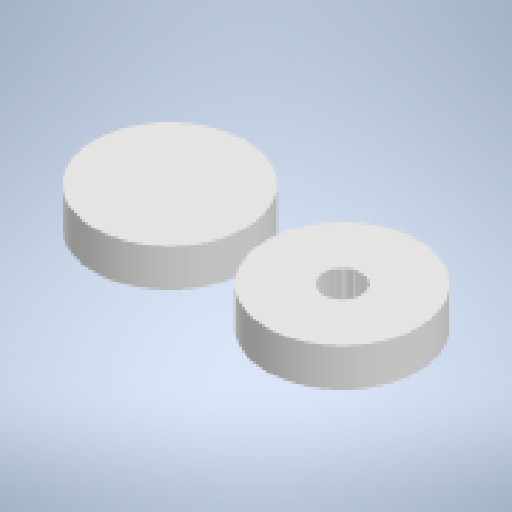
# Autodesk Inventor part: klesce2
Saved by Autodesk Inventor 2024 (Build 280153000, 153)
## iProperties
Created: 2023-09-14
Part Number: klesce2
Material: Generic
Document SubType Name: Modeling
Designer: jebes windows
Density: 1 g/cm^3
Appearance: Default
Author: jebes windows
Autodesk Inventor part; units mm, degrees
ref_plane "YZ Plane" through (0, 0, 0) normal (1, 0, 0) x (0, 1, 0)
ref_plane "XZ Plane" through (0, 0, 0) normal (0, 1, 0) x (-1, 0, 0)
ref_plane "XY Plane" through (0, 0, 0) normal (0, 0, 1) x (1, 0, 0)
sketch "Sketch1" plane through (0, 0, 0) normal (0, 0, 1) x (1, 0, 0)
  circle A0 centre (0, 0) radius 2.25 projected
  circle A1 centre (0, 0) radius 0.8 projected
  line L0 (-1.3596, 2.0381) -> (-1.3813, 1.9012) projected
  arc A2 (-1.3089, 2.071) -> (-1.3596, 2.0381) centre (0, 0) ccw projected
  line L1 (-1.175, 2.0352) -> (-1.3089, 2.071) projected
  line L2 (-1.1391, 2.1691) -> (-1.175, 2.0352) projected
  arc A3 (-1.0853, 2.1965) -> (-1.1391, 2.1691) centre (0, 0) ccw projected
  line L3 (-0.9558, 2.1468) -> (-1.0853, 2.1965) projected
  circle A4 centre (0, 0) radius 2.5 projected
  circle A5 centre (0, 0) radius 0.8 projected
  line L4 (-0.9061, 2.2763) -> (-0.9558, 2.1468) projected
  arc A6 (-0.8497, 2.2979) -> (-0.9061, 2.2763) centre (0, 0) ccw projected
  line L5 (-0.7262, 2.235) -> (-0.8497, 2.2979) projected
  line L6 (-0.6632, 2.3585) -> (-0.7262, 2.235) projected
  arc A7 (-0.6049, 2.3742) -> (-0.6632, 2.3585) centre (0, 0) ccw projected
  line L7 (-0.4886, 2.2986) -> (-0.6049, 2.3742) projected
  line L8 (-0.4131, 2.4149) -> (-0.4886, 2.2986) projected
  arc A8 (-0.3534, 2.4244) -> (-0.4131, 2.4149) centre (0, 0) ccw projected
  line L9 (-0.2456, 2.3371) -> (-0.3534, 2.4244) projected
  line L10 (-0.1584, 2.4449) -> (-0.2456, 2.3371) projected
  arc A9 (-0.098, 2.448) -> (-0.1584, 2.4449) centre (0, 0) ccw projected
  line L11 (0, 2.35) -> (-0.098, 2.448) projected
  line L12 (-1.5652, 1.8848) -> (-1.5725, 1.7464) projected
  line L13 (-1.3813, 1.9012) -> (-1.5182, 1.9229) projected
  arc A10 (-1.5182, 1.9229) -> (-1.5652, 1.8848) centre (0, 0) ccw projected
  line L14 (-1.5725, 1.7464) -> (-1.7109, 1.7536) projected
  arc A11 (-1.7109, 1.7536) -> (-1.7536, 1.7109) centre (0, 0) ccw projected
  line L15 (-1.7536, 1.7109) -> (-1.7464, 1.5725) projected
  line L16 (-1.7464, 1.5725) -> (-1.8848, 1.5652) projected
  arc A12 (-1.8848, 1.5652) -> (-1.9229, 1.5182) centre (0, 0) ccw projected
  line L17 (-1.9229, 1.5182) -> (-1.9012, 1.3813) projected
  line L18 (-1.9012, 1.3813) -> (-2.0381, 1.3596) projected
  arc A13 (-2.0381, 1.3596) -> (-2.071, 1.3089) centre (0, 0) ccw projected
  line L19 (-2.071, 1.3089) -> (-2.0352, 1.175) projected
  line L20 (-2.0352, 1.175) -> (-2.1691, 1.1391) projected
  arc A14 (-2.1691, 1.1391) -> (-2.1965, 1.0853) centre (0, 0) ccw projected
  line L21 (-2.1965, 1.0853) -> (-2.1468, 0.9558) projected
  circle A15 centre (0, 0) radius 2.5 projected
  circle A16 centre (0, 0) radius 0.8 projected
  line L22 (-2.1468, 0.9558) -> (-2.2763, 0.9061) projected
  arc A17 (-2.2763, 0.9061) -> (-2.2979, 0.8497) centre (0, 0) ccw projected
  line L23 (-2.2979, 0.8497) -> (-2.235, 0.7262) projected
  line L24 (-2.235, 0.7262) -> (-2.3585, 0.6632) projected
  arc A18 (-2.3585, 0.6632) -> (-2.3742, 0.6049) centre (0, 0) ccw projected
  line L25 (-2.3742, 0.6049) -> (-2.2986, 0.4886) projected
  line L26 (-2.2986, 0.4886) -> (-2.4149, 0.4131) projected
  arc A19 (-2.4149, 0.4131) -> (-2.4244, 0.3534) centre (0, 0) ccw projected
  circle A20 centre (0, 0) radius 2.5 projected
  circle A21 centre (0, 0) radius 0.8 projected
  line L27 (-2.4244, 0.3534) -> (-2.3371, 0.2456) projected
  circle A22 centre (0, 0) radius 2.5 projected
  circle A23 centre (0, 0) radius 0.8 projected
  line L28 (-2.3371, 0.2456) -> (-2.4449, 0.1584) projected
  arc A24 (-2.4449, 0.1584) -> (-2.448, 0.098) centre (0, 0) ccw projected
  circle A25 centre (0, 0) radius 2.5 projected
  circle A26 centre (0, 0) radius 0.8 projected
  line L29 (-2.448, 0.098) -> (-2.35, 0) projected
  line L30 (0.098, 2.448) -> (0, 2.35) projected
  arc A27 (0.1584, 2.4449) -> (0.098, 2.448) centre (0, 0) ccw projected
  line L31 (0.2456, 2.3371) -> (0.1584, 2.4449) projected
  line L32 (0.3534, 2.4244) -> (0.2456, 2.3371) projected
  arc A28 (0.4131, 2.4149) -> (0.3534, 2.4244) centre (0, 0) ccw projected
  line L33 (0.4886, 2.2986) -> (0.4131, 2.4149) projected
  line L34 (0.6049, 2.3742) -> (0.4886, 2.2986) projected
  line L35 (0.7262, 2.235) -> (0.6632, 2.3585) projected
  arc A29 (0.6632, 2.3585) -> (0.6049, 2.3742) centre (0, 0) ccw projected
  line L36 (0.8497, 2.2979) -> (0.7262, 2.235) projected
  line L37 (0.9558, 2.1468) -> (0.9061, 2.2763) projected
  arc A30 (0.9061, 2.2763) -> (0.8497, 2.2979) centre (0, 0) ccw projected
  line L38 (1.0853, 2.1965) -> (0.9558, 2.1468) projected
  line L39 (1.175, 2.0352) -> (1.1391, 2.1691) projected
  arc A31 (1.1391, 2.1691) -> (1.0853, 2.1965) centre (0, 0) ccw projected
  line L40 (1.3089, 2.071) -> (1.175, 2.0352) projected
  arc A32 (1.3596, 2.0381) -> (1.3089, 2.071) centre (0, 0) ccw projected
  line L41 (1.3813, 1.9012) -> (1.3596, 2.0381) projected
  line L42 (1.5182, 1.9229) -> (1.3813, 1.9012) projected
  arc A33 (1.5652, 1.8848) -> (1.5182, 1.9229) centre (0, 0) ccw projected
  line L43 (1.5725, 1.7464) -> (1.5652, 1.8848) projected
  line L44 (1.7109, 1.7536) -> (1.5725, 1.7464) projected
  line L45 (1.7464, 1.5725) -> (1.7536, 1.7109) projected
  arc A34 (1.7536, 1.7109) -> (1.7109, 1.7536) centre (0, 0) ccw projected
  line L46 (1.8848, 1.5652) -> (1.7464, 1.5725) projected
  arc A35 (1.9229, 1.5182) -> (1.8848, 1.5652) centre (0, 0) ccw projected
  line L47 (1.9012, 1.3813) -> (1.9229, 1.5182) projected
  line L48 (2.0381, 1.3596) -> (1.9012, 1.3813) projected
  arc A36 (2.071, 1.3089) -> (2.0381, 1.3596) centre (0, 0) ccw projected
  line L49 (2.0352, 1.175) -> (2.071, 1.3089) projected
  line L50 (2.1691, 1.1391) -> (2.0352, 1.175) projected
  arc A37 (2.1965, 1.0853) -> (2.1691, 1.1391) centre (0, 0) ccw projected
  line L51 (2.1468, 0.9558) -> (2.1965, 1.0853) projected
  line L52 (2.2763, 0.9061) -> (2.1468, 0.9558) projected
  circle A38 centre (0, 0) radius 2.5 projected
  circle A39 centre (0, 0) radius 0.8 projected
  arc A40 (2.2979, 0.8497) -> (2.2763, 0.9061) centre (0, 0) ccw projected
  line L53 (2.235, 0.7262) -> (2.2979, 0.8497) projected
  line L54 (2.3585, 0.6632) -> (2.235, 0.7262) projected
  arc A41 (2.3742, 0.6049) -> (2.3585, 0.6632) centre (0, 0) ccw projected
  line L55 (2.2986, 0.4886) -> (2.3742, 0.6049) projected
  line L56 (2.4149, 0.4131) -> (2.2986, 0.4886) projected
  circle A42 centre (0, 0) radius 2.5 projected
  circle A43 centre (0, 0) radius 0.8 projected
  arc A44 (2.4244, 0.3534) -> (2.4149, 0.4131) centre (0, 0) ccw projected
  circle A45 centre (0, 0) radius 2.5 projected
  circle A46 centre (0, 0) radius 0.8 projected
  line L57 (2.3371, 0.2456) -> (2.4244, 0.3534) projected
  line L58 (2.4449, 0.1584) -> (2.3371, 0.2456) projected
  circle A47 centre (0, 0) radius 2.5 projected
  circle A48 centre (0, 0) radius 0.8 projected
  arc A49 (2.448, 0.098) -> (2.4449, 0.1584) centre (0, 0) ccw projected
  line L59 (2.35, 0) -> (2.448, 0.098) projected
  line L60 (2.448, -0.098) -> (2.35, 0) projected
  line L61 (2.3371, -0.2456) -> (2.4449, -0.1584) projected
  arc A50 (2.4449, -0.1584) -> (2.448, -0.098) centre (0, 0) ccw projected
  line L62 (2.4244, -0.3534) -> (2.3371, -0.2456) projected
  arc A51 (2.4149, -0.4131) -> (2.4244, -0.3534) centre (0, 0) ccw projected
  circle A52 centre (0, 0) radius 2.5 projected
  circle A53 centre (0, 0) radius 0.8 projected
  line L63 (2.2986, -0.4886) -> (2.4149, -0.4131) projected
  circle A54 centre (0, 0) radius 2.5 projected
  circle A55 centre (0, 0) radius 0.8 projected
  line L64 (2.3742, -0.6049) -> (2.2986, -0.4886) projected
  circle A56 centre (0, 0) radius 2.5 projected
  circle A57 centre (0, 0) radius 0.8 projected
  arc A58 (2.3585, -0.6632) -> (2.3742, -0.6049) centre (0, 0) ccw projected
  line L65 (2.235, -0.7262) -> (2.3585, -0.6632) projected
  circle A59 centre (0, 0) radius 2.5 projected
  circle A60 centre (0, 0) radius 0.8 projected
  line L66 (2.2979, -0.8497) -> (2.235, -0.7262) projected
  arc A61 (2.2763, -0.9061) -> (2.2979, -0.8497) centre (0, 0) ccw projected
  circle A62 centre (0, 0) radius 2.5 projected
  circle A63 centre (0, 0) radius 0.8 projected
  line L67 (2.1468, -0.9558) -> (2.2763, -0.9061) projected
  line L68 (2.1965, -1.0853) -> (2.1468, -0.9558) projected
  circle A64 centre (0, 0) radius 2.5 projected
  circle A65 centre (0, 0) radius 0.8 projected
  arc A66 (2.1691, -1.1391) -> (2.1965, -1.0853) centre (0, 0) ccw projected
  line L69 (2.0352, -1.175) -> (2.1691, -1.1391) projected
  circle A67 centre (0, 0) radius 2.5 projected
  circle A68 centre (0, 0) radius 0.8 projected
  circle A69 centre (0, 0) radius 2.5 projected
  circle A70 centre (0, 0) radius 0.8 projected
  line L70 (2.071, -1.3089) -> (2.0352, -1.175) projected
  arc A71 (2.0381, -1.3596) -> (2.071, -1.3089) centre (0, 0) ccw projected
  line L71 (1.9012, -1.3813) -> (2.0381, -1.3596) projected
  circle A72 centre (0, 0) radius 2.5 projected
  circle A73 centre (0, 0) radius 0.8 projected
  line L72 (1.9229, -1.5182) -> (1.9012, -1.3813) projected
  circle A74 centre (0, 0) radius 2.5 projected
  circle A75 centre (0, 0) radius 0.8 projected
  arc A76 (1.8848, -1.5652) -> (1.9229, -1.5182) centre (0, 0) ccw projected
  circle A77 centre (0, 0) radius 2.5 projected
  circle A78 centre (0, 0) radius 0.8 projected
  circle A79 centre (0, 0) radius 2.5 projected
  circle A80 centre (0, 0) radius 0.8 projected
  line L73 (1.7536, -1.7109) -> (1.7464, -1.5725) projected
  line L74 (1.7536, -1.7109) -> (1.7464, -1.5725) projected
  line L75 (1.7536, -1.7109) -> (1.7464, -1.5725) projected
  line L76 (1.7464, -1.5725) -> (1.8848, -1.5652) projected
  arc A81 (1.7109, -1.7536) -> (1.7536, -1.7109) centre (0, 0) ccw projected
  line L77 (1.5725, -1.7464) -> (1.7109, -1.7536) projected
  circle A82 centre (0, 0) radius 2.5 projected
  circle A83 centre (0, 0) radius 0.8 projected
  line L78 (1.5652, -1.8848) -> (1.5725, -1.7464) projected
  arc A84 (1.5182, -1.9229) -> (1.5652, -1.8848) centre (0, 0) ccw projected
  circle A85 centre (0, 0) radius 2.5 projected
  circle A86 centre (0, 0) radius 0.8 projected
  line L79 (1.3813, -1.9012) -> (1.5182, -1.9229) projected
  circle A87 centre (0, 0) radius 2.5 projected
  circle A88 centre (0, 0) radius 0.8 projected
  line L80 (1.3596, -2.0381) -> (1.3813, -1.9012) projected
  arc A89 (1.3089, -2.071) -> (1.3596, -2.0381) centre (0, 0) ccw projected
  circle A90 centre (0, 0) radius 2.5 projected
  circle A91 centre (0, 0) radius 0.8 projected
  line L81 (1.175, -2.0352) -> (1.3089, -2.071) projected
  line L82 (1.1391, -2.1691) -> (1.175, -2.0352) projected
  arc A92 (1.0853, -2.1965) -> (1.1391, -2.1691) centre (0, 0) ccw projected
  line L83 (0.9558, -2.1468) -> (1.0853, -2.1965) projected
  line L84 (0.9061, -2.2763) -> (0.9558, -2.1468) projected
  arc A93 (0.8497, -2.2979) -> (0.9061, -2.2763) centre (0, 0) ccw projected
  line L85 (0.7262, -2.235) -> (0.8497, -2.2979) projected
  line L86 (0.6632, -2.3585) -> (0.7262, -2.235) projected
  arc A94 (0.6049, -2.3742) -> (0.6632, -2.3585) centre (0, 0) ccw projected
  line L87 (0.4886, -2.2986) -> (0.6049, -2.3742) projected
  circle A95 centre (0, 0) radius 2.5 projected
  circle A96 centre (0, 0) radius 0.8 projected
  circle A97 centre (0, 0) radius 2.5 projected
  circle A98 centre (0, 0) radius 0.8 projected
  line L88 (0.4131, -2.4149) -> (0.4886, -2.2986) projected
  arc A99 (0.3534, -2.4244) -> (0.4131, -2.4149) centre (0, 0) ccw projected
  line L89 (0.2456, -2.3371) -> (0.3534, -2.4244) projected
  line L90 (0.1584, -2.4449) -> (0.2456, -2.3371) projected
  arc A100 (0.098, -2.448) -> (0.1584, -2.4449) centre (0, 0) ccw projected
  circle A101 centre (0, 0) radius 2.5 projected
  circle A102 centre (0, 0) radius 0.8 projected
  line L91 (0, -2.35) -> (0.098, -2.448) projected
  circle A103 centre (0, 0) radius 2.5 projected
  circle A104 centre (0, 0) radius 0.8 projected
  line L92 (-0.098, -2.448) -> (0, -2.35) projected
  arc A105 (-0.1584, -2.4449) -> (-0.098, -2.448) centre (0, 0) ccw projected
  circle A106 centre (0, 0) radius 2.5 projected
  circle A107 centre (0, 0) radius 0.8 projected
  circle A108 centre (0, 0) radius 2.5 projected
  circle A109 centre (0, 0) radius 0.8 projected
  circle A110 centre (0, 0) radius 2.5 projected
  circle A111 centre (0, 0) radius 0.8 projected
  line L93 (-0.2456, -2.3371) -> (-0.1584, -2.4449) projected
  line L94 (-0.3534, -2.4244) -> (-0.2456, -2.3371) projected
  circle A112 centre (0, 0) radius 2.5 projected
  circle A113 centre (0, 0) radius 0.8 projected
  arc A114 (-0.4131, -2.4149) -> (-0.3534, -2.4244) centre (0, 0) ccw projected
  line L95 (-0.4886, -2.2986) -> (-0.4131, -2.4149) projected
  line L96 (-0.6049, -2.3742) -> (-0.4886, -2.2986) projected
  arc A115 (-0.6632, -2.3585) -> (-0.6049, -2.3742) centre (0, 0) ccw projected
  line L97 (-0.7262, -2.235) -> (-0.6632, -2.3585) projected
  line L98 (-0.8497, -2.2979) -> (-0.7262, -2.235) projected
  arc A116 (-0.9061, -2.2763) -> (-0.8497, -2.2979) centre (0, 0) ccw projected
  circle A117 centre (0, 0) radius 2.5 projected
  circle A118 centre (0, 0) radius 0.8 projected
  line L99 (-0.9558, -2.1468) -> (-0.9061, -2.2763) projected
  line L100 (-1.0853, -2.1965) -> (-0.9558, -2.1468) projected
  arc A119 (-1.1391, -2.1691) -> (-1.0853, -2.1965) centre (0, 0) ccw projected
  line L101 (-1.175, -2.0352) -> (-1.1391, -2.1691) projected
  line L102 (-1.3089, -2.071) -> (-1.175, -2.0352) projected
  arc A120 (-1.3596, -2.0381) -> (-1.3089, -2.071) centre (0, 0) ccw projected
  circle A121 centre (0, 0) radius 2.5 projected
  circle A122 centre (0, 0) radius 0.8 projected
  line L103 (-1.3813, -1.9012) -> (-1.3596, -2.0381) projected
  line L104 (-1.5182, -1.9229) -> (-1.3813, -1.9012) projected
  arc A123 (-1.5652, -1.8848) -> (-1.5182, -1.9229) centre (0, 0) ccw projected
  line L105 (-1.5725, -1.7464) -> (-1.5652, -1.8848) projected
  circle A124 centre (0, 0) radius 2.5 projected
  circle A125 centre (0, 0) radius 0.8 projected
  line L106 (-1.7109, -1.7536) -> (-1.5725, -1.7464) projected
  arc A126 (-1.7536, -1.7109) -> (-1.7109, -1.7536) centre (0, 0) ccw projected
  circle A127 centre (0, 0) radius 2.5 projected
  circle A128 centre (0, 0) radius 0.8 projected
  line L107 (-1.7464, -1.5725) -> (-1.7536, -1.7109) projected
  line L108 (-1.8848, -1.5652) -> (-1.7464, -1.5725) projected
  arc A129 (-1.9229, -1.5182) -> (-1.8848, -1.5652) centre (0, 0) ccw projected
  circle A130 centre (0, 0) radius 2.5 projected
  circle A131 centre (0, 0) radius 0.8 projected
  line L109 (-1.9012, -1.3813) -> (-1.9229, -1.5182) projected
  circle A132 centre (0, 0) radius 2.5 projected
  circle A133 centre (0, 0) radius 0.8 projected
  line L110 (-2.0381, -1.3596) -> (-1.9012, -1.3813) projected
  arc A134 (-2.071, -1.3089) -> (-2.0381, -1.3596) centre (0, 0) ccw projected
  line L111 (-2.0352, -1.175) -> (-2.071, -1.3089) projected
  line L112 (-2.1691, -1.1391) -> (-2.0352, -1.175) projected
  arc A135 (-2.1965, -1.0853) -> (-2.1691, -1.1391) centre (0, 0) ccw projected
  line L113 (-2.1468, -0.9558) -> (-2.1965, -1.0853) projected
  circle A136 centre (0, 0) radius 2.5 projected
  circle A137 centre (0, 0) radius 0.8 projected
  line L114 (-2.2763, -0.9061) -> (-2.1468, -0.9558) projected
  arc A138 (-2.2979, -0.8497) -> (-2.2763, -0.9061) centre (0, 0) ccw projected
  line L115 (-2.235, -0.7262) -> (-2.2979, -0.8497) projected
  line L116 (-2.3585, -0.6632) -> (-2.235, -0.7262) projected
  arc A139 (-2.3742, -0.6049) -> (-2.3585, -0.6632) centre (0, 0) ccw projected
  line L117 (-2.2986, -0.4886) -> (-2.3742, -0.6049) projected
  circle A140 centre (0, 0) radius 2.5 projected
  circle A141 centre (0, 0) radius 0.8 projected
  line L118 (-2.4149, -0.4131) -> (-2.2986, -0.4886) projected
  arc A142 (-2.4244, -0.3534) -> (-2.4149, -0.4131) centre (0, 0) ccw projected
  line L119 (-2.3371, -0.2456) -> (-2.4244, -0.3534) projected
  line L120 (-2.4449, -0.1584) -> (-2.3371, -0.2456) projected
  arc A143 (-2.448, -0.098) -> (-2.4449, -0.1584) centre (0, 0) ccw projected
  line L121 (-2.35, 0) -> (-2.448, -0.098) projected
  line L122 (-2.448, 0.098) -> (-2.35, 0) projected
  arc A144 (-2.4933, 0.1836) -> (-2.498, 0.1) centre (0, 0) ccw
  line L123 (-2.4933, 0.1836) -> (-2.4074, 0.253)
  line L124 (-2.4074, 0.253) -> (-2.4769, 0.3388)
  arc A145 (-2.4604, 0.4432) -> (-2.4769, 0.3388) centre (0, 0) ccw
  line L125 (-2.4604, 0.4432) -> (-2.3678, 0.5033)
  line L126 (-2.3678, 0.5033) -> (-2.4279, 0.5959)
  arc A146 (-2.4006, 0.6979) -> (-2.4279, 0.5959) centre (0, 0) ccw
  line L127 (-2.4006, 0.6979) -> (-2.3022, 0.748)
  line L128 (-2.3022, 0.748) -> (-2.3524, 0.8464)
  arc A147 (-2.3145, 0.945) -> (-2.3524, 0.8464) centre (0, 0) ccw
  line L129 (-2.3145, 0.945) -> (-2.2114, 0.9846)
  line L130 (-2.2114, 0.9846) -> (-2.251, 1.0877)
  arc A148 (-2.203, 1.1818) -> (-2.251, 1.0877) centre (0, 0) ccw
  line L131 (-2.203, 1.1818) -> (-2.0964, 1.2104)
  line L132 (-2.0964, 1.2104) -> (-2.125, 1.317)
  arc A149 (-2.0674, 1.4056) -> (-2.125, 1.317) centre (0, 0) ccw
  line L133 (-2.0674, 1.4056) -> (-1.9584, 1.4229)
  line L134 (-1.9584, 1.4229) -> (-1.9757, 1.5319)
  arc A150 (-1.9092, 1.614) -> (-1.9757, 1.5319) centre (0, 0) ccw
  line L135 (-1.9092, 1.614) -> (-1.7989, 1.6198)
  line L136 (-1.7989, 1.6198) -> (-1.8047, 1.73)
  arc A151 (-1.73, 1.8047) -> (-1.8047, 1.73) centre (0, 0) ccw
  line L137 (-1.73, 1.8047) -> (-1.6198, 1.7989)
  line L138 (-1.6198, 1.7989) -> (-1.614, 1.9092)
  arc A152 (-1.5319, 1.9757) -> (-1.614, 1.9092) centre (0, 0) ccw
  line L139 (-1.5319, 1.9757) -> (-1.4229, 1.9584)
  line L140 (-1.4229, 1.9584) -> (-1.4056, 2.0674)
  arc A153 (-1.317, 2.125) -> (-1.4056, 2.0674) centre (0, 0) ccw
  line L141 (-1.317, 2.125) -> (-1.2104, 2.0964)
  line L142 (-1.2104, 2.0964) -> (-1.1818, 2.203)
  arc A154 (-1.0877, 2.251) -> (-1.1818, 2.203) centre (0, 0) ccw
  line L143 (-1.0877, 2.251) -> (-0.9846, 2.2114)
  line L144 (-0.9846, 2.2114) -> (-0.945, 2.3145)
  arc A155 (-0.8464, 2.3524) -> (-0.945, 2.3145) centre (0, 0) ccw
  line L145 (-0.8464, 2.3524) -> (-0.748, 2.3022)
  line L146 (-0.748, 2.3022) -> (-0.6979, 2.4006)
  arc A156 (-0.5959, 2.4279) -> (-0.6979, 2.4006) centre (0, 0) ccw
  line L147 (-0.5959, 2.4279) -> (-0.5033, 2.3678)
  line L148 (-0.5033, 2.3678) -> (-0.4432, 2.4604)
  arc A157 (-0.3388, 2.4769) -> (-0.4432, 2.4604) centre (0, 0) ccw
  line L149 (-0.3388, 2.4769) -> (-0.253, 2.4074)
  line L150 (-0.253, 2.4074) -> (-0.1836, 2.4933)
  arc A158 (-0.0781, 2.4988) -> (-0.1836, 2.4933) centre (0, 0) ccw
  line L151 (-0.0781, 2.4988) -> (0, 2.4207)
  line L152 (0, 2.4207) -> (0.0781, 2.4988)
  arc A159 (0.1836, 2.4933) -> (0.0781, 2.4988) centre (0, 0) ccw
  line L153 (0.1836, 2.4933) -> (0.253, 2.4074)
  line L154 (0.253, 2.4074) -> (0.3388, 2.4769)
  arc A160 (0.4432, 2.4604) -> (0.3388, 2.4769) centre (0, 0) ccw
  line L155 (0.4432, 2.4604) -> (0.5033, 2.3678)
  line L156 (0.5033, 2.3678) -> (0.5959, 2.4279)
  arc A161 (0.6979, 2.4006) -> (0.5959, 2.4279) centre (0, 0) ccw
  line L157 (0.6979, 2.4006) -> (0.748, 2.3022)
  line L158 (0.748, 2.3022) -> (0.8464, 2.3524)
  arc A162 (0.945, 2.3145) -> (0.8464, 2.3524) centre (0, 0) ccw
  line L159 (0.945, 2.3145) -> (0.9846, 2.2114)
  line L160 (0.9846, 2.2114) -> (1.0877, 2.251)
  arc A163 (1.1818, 2.203) -> (1.0877, 2.251) centre (0, 0) ccw
  line L161 (1.1818, 2.203) -> (1.2104, 2.0964)
  line L162 (1.2104, 2.0964) -> (1.317, 2.125)
  arc A164 (1.4056, 2.0674) -> (1.317, 2.125) centre (0, 0) ccw
  line L163 (1.4056, 2.0674) -> (1.4229, 1.9584)
  line L164 (1.4229, 1.9584) -> (1.5319, 1.9757)
  arc A165 (1.614, 1.9092) -> (1.5319, 1.9757) centre (0, 0) ccw
  line L165 (1.614, 1.9092) -> (1.6198, 1.7989)
  line L166 (1.6198, 1.7989) -> (1.73, 1.8047)
  arc A166 (1.8047, 1.73) -> (1.73, 1.8047) centre (0, 0) ccw
  line L167 (1.8047, 1.73) -> (1.7989, 1.6198)
  line L168 (1.7989, 1.6198) -> (1.9092, 1.614)
  arc A167 (1.9757, 1.5319) -> (1.9092, 1.614) centre (0, 0) ccw
  line L169 (1.9757, 1.5319) -> (1.9584, 1.4229)
  line L170 (1.9584, 1.4229) -> (2.0674, 1.4056)
  arc A168 (2.125, 1.317) -> (2.0674, 1.4056) centre (0, 0) ccw
  line L171 (2.125, 1.317) -> (2.0964, 1.2104)
  line L172 (2.0964, 1.2104) -> (2.203, 1.1818)
  arc A169 (2.251, 1.0877) -> (2.203, 1.1818) centre (0, 0) ccw
  line L173 (2.251, 1.0877) -> (2.2114, 0.9846)
  line L174 (2.2114, 0.9846) -> (2.3145, 0.945)
  arc A170 (2.3524, 0.8464) -> (2.3145, 0.945) centre (0, 0) ccw
  line L175 (2.3524, 0.8464) -> (2.3022, 0.748)
  line L176 (2.3022, 0.748) -> (2.4006, 0.6979)
  arc A171 (2.4279, 0.5959) -> (2.4006, 0.6979) centre (0, 0) ccw
  line L177 (2.4279, 0.5959) -> (2.3678, 0.5033)
  line L178 (2.3678, 0.5033) -> (2.4604, 0.4432)
  arc A172 (2.4769, 0.3388) -> (2.4604, 0.4432) centre (0, 0) ccw
  line L179 (2.4769, 0.3388) -> (2.4074, 0.253)
  line L180 (2.4074, 0.253) -> (2.4933, 0.1836)
  arc A173 (2.4988, 0.0781) -> (2.4933, 0.1836) centre (0, 0) ccw
  line L181 (2.4988, 0.0781) -> (2.4207, 0)
  line L182 (2.4207, 0) -> (2.4988, -0.0781)
  arc A174 (2.4933, -0.1836) -> (2.4988, -0.0781) centre (0, 0) ccw
  line L183 (2.4933, -0.1836) -> (2.4074, -0.253)
  line L184 (2.4074, -0.253) -> (2.4769, -0.3388)
  arc A175 (2.4604, -0.4432) -> (2.4769, -0.3388) centre (0, 0) ccw
  line L185 (2.4604, -0.4432) -> (2.3678, -0.5033)
  line L186 (2.3678, -0.5033) -> (2.4279, -0.5959)
  arc A176 (2.4006, -0.6979) -> (2.4279, -0.5959) centre (0, 0) ccw
  line L187 (2.4006, -0.6979) -> (2.3022, -0.748)
  line L188 (2.3022, -0.748) -> (2.3524, -0.8464)
  arc A177 (2.3145, -0.945) -> (2.3524, -0.8464) centre (0, 0) ccw
  line L189 (2.3145, -0.945) -> (2.2114, -0.9846)
  line L190 (2.2114, -0.9846) -> (2.251, -1.0877)
  arc A178 (2.203, -1.1818) -> (2.251, -1.0877) centre (0, 0) ccw
  line L191 (2.203, -1.1818) -> (2.0964, -1.2104)
  line L192 (2.0964, -1.2104) -> (2.125, -1.317)
  arc A179 (2.0674, -1.4056) -> (2.125, -1.317) centre (0, 0) ccw
  line L193 (2.0674, -1.4056) -> (1.9584, -1.4229)
  line L194 (1.9584, -1.4229) -> (1.9757, -1.5319)
  arc A180 (1.9092, -1.614) -> (1.9757, -1.5319) centre (0, 0) ccw
  line L195 (1.9092, -1.614) -> (1.749, -1.6224)
  arc A181 (1.73, -1.8047) -> (1.7894, -1.7458) centre (0, 0) ccw
  line L196 (1.73, -1.8047) -> (1.6198, -1.7989)
  line L197 (1.6198, -1.7989) -> (1.614, -1.9092)
  arc A182 (1.5319, -1.9757) -> (1.614, -1.9092) centre (0, 0) ccw
  line L198 (1.5319, -1.9757) -> (1.4229, -1.9584)
  line L199 (1.4229, -1.9584) -> (1.4056, -2.0674)
  arc A183 (1.317, -2.125) -> (1.4056, -2.0674) centre (0, 0) ccw
  line L200 (1.317, -2.125) -> (1.2104, -2.0964)
  line L201 (1.2104, -2.0964) -> (1.1818, -2.203)
  arc A184 (1.0877, -2.251) -> (1.1818, -2.203) centre (0, 0) ccw
  line L202 (1.0877, -2.251) -> (0.9846, -2.2114)
  line L203 (0.9846, -2.2114) -> (0.945, -2.3145)
  arc A185 (0.8464, -2.3524) -> (0.945, -2.3145) centre (0, 0) ccw
  line L204 (0.8464, -2.3524) -> (0.748, -2.3022)
  line L205 (0.748, -2.3022) -> (0.6979, -2.4006)
  arc A186 (0.5959, -2.4279) -> (0.6979, -2.4006) centre (0, 0) ccw
  line L206 (0.5959, -2.4279) -> (0.5033, -2.3678)
  line L207 (0.5033, -2.3678) -> (0.4432, -2.4604)
  arc A187 (0.3388, -2.4769) -> (0.4432, -2.4604) centre (0, 0) ccw
  line L208 (0.3388, -2.4769) -> (0.253, -2.4074)
  line L209 (0.253, -2.4074) -> (0.1836, -2.4933)
  arc A188 (0.0781, -2.4988) -> (0.1836, -2.4933) centre (0, 0) ccw
  line L210 (0.0781, -2.4988) -> (0, -2.4207)
  line L211 (0, -2.4207) -> (-0.0781, -2.4988)
  arc A189 (-0.1836, -2.4933) -> (-0.0781, -2.4988) centre (0, 0) ccw
  line L212 (-0.1836, -2.4933) -> (-0.253, -2.4074)
  line L213 (-0.253, -2.4074) -> (-0.3388, -2.4769)
  arc A190 (-0.4432, -2.4604) -> (-0.3388, -2.4769) centre (0, 0) ccw
  line L214 (-0.4432, -2.4604) -> (-0.5033, -2.3678)
  line L215 (-0.5033, -2.3678) -> (-0.5959, -2.4279)
  arc A191 (-0.6979, -2.4006) -> (-0.5959, -2.4279) centre (0, 0) ccw
  line L216 (-0.6979, -2.4006) -> (-0.748, -2.3022)
  line L217 (-0.748, -2.3022) -> (-0.8464, -2.3524)
  arc A192 (-0.945, -2.3145) -> (-0.8464, -2.3524) centre (0, 0) ccw
  line L218 (-0.945, -2.3145) -> (-0.9846, -2.2114)
  line L219 (-0.9846, -2.2114) -> (-1.0877, -2.251)
  arc A193 (-1.1818, -2.203) -> (-1.0877, -2.251) centre (0, 0) ccw
  line L220 (-1.1818, -2.203) -> (-1.2104, -2.0964)
  line L221 (-1.2104, -2.0964) -> (-1.317, -2.125)
  arc A194 (-1.4056, -2.0674) -> (-1.317, -2.125) centre (0, 0) ccw
  line L222 (-1.4056, -2.0674) -> (-1.4229, -1.9584)
  line L223 (-1.4229, -1.9584) -> (-1.5319, -1.9757)
  arc A195 (-1.614, -1.9092) -> (-1.5319, -1.9757) centre (0, 0) ccw
  line L224 (-1.614, -1.9092) -> (-1.6198, -1.7989)
  line L225 (-1.6198, -1.7989) -> (-1.73, -1.8047)
  arc A196 (-1.8047, -1.73) -> (-1.73, -1.8047) centre (0, 0) ccw
  line L226 (-1.8047, -1.73) -> (-1.7989, -1.6198)
  line L227 (-1.7989, -1.6198) -> (-1.9092, -1.614)
  arc A197 (-1.9757, -1.5319) -> (-1.9092, -1.614) centre (0, 0) ccw
  line L228 (-1.9757, -1.5319) -> (-1.9584, -1.4229)
  line L229 (-1.9584, -1.4229) -> (-2.0674, -1.4056)
  arc A198 (-2.125, -1.317) -> (-2.0674, -1.4056) centre (0, 0) ccw
  line L230 (-2.125, -1.317) -> (-2.0964, -1.2104)
  line L231 (-2.0964, -1.2104) -> (-2.203, -1.1818)
  arc A199 (-2.251, -1.0877) -> (-2.203, -1.1818) centre (0, 0) ccw
  line L232 (-2.251, -1.0877) -> (-2.2114, -0.9846)
  line L233 (-2.2114, -0.9846) -> (-2.3145, -0.945)
  arc A200 (-2.3524, -0.8464) -> (-2.3145, -0.945) centre (0, 0) ccw
  line L234 (-2.3524, -0.8464) -> (-2.3022, -0.748)
  line L235 (-2.3022, -0.748) -> (-2.4006, -0.6979)
  arc A201 (-2.4279, -0.5959) -> (-2.4006, -0.6979) centre (0, 0) ccw
  line L236 (-2.4279, -0.5959) -> (-2.3678, -0.5033)
  line L237 (-2.3678, -0.5033) -> (-2.4604, -0.4432)
  arc A202 (-2.4769, -0.3388) -> (-2.4604, -0.4432) centre (0, 0) ccw
  line L238 (-2.4769, -0.3388) -> (-2.4074, -0.253)
  line L239 (-2.4074, -0.253) -> (-2.4933, -0.1836)
  arc A203 (-2.4988, -0.0781) -> (-2.4933, -0.1836) centre (0, 0) ccw
  line L240 (-2.4988, -0.0781) -> (-2.3854, 0.0354)
  line L241 (1.8047, -1.73) -> (1.7963, -1.5698)
  line L242 (1.7894, -1.7458) -> (1.8047, -1.73)
  line L243 (-2.4988, 0.0781) -> (-2.3854, -0.0354)
  line L244 (-2.4988, 0.0781) -> (-2.498, 0.1)
  circle A204 centre (0, 0) radius 10
  point P0 (0, 0)
  point P1 (2.4933, -0.1836)
  point P2 (2.4604, -0.4432)
  point P3 (2.4006, -0.6979)
  point P4 (2.3145, -0.945)
  point P5 (2.203, -1.1818)
  point P6 (2.0674, -1.4056)
  point P7 (1.9092, -1.614)
  point P8 (1.7989, -1.6198)
  point P9 (1.73, -1.8047)
  point P10 (1.5319, -1.9757)
  point P11 (1.317, -2.125)
  point P12 (1.0877, -2.251)
  point P13 (0.8464, -2.3524)
  point P14 (0.5959, -2.4279)
  point P15 (0.3388, -2.4769)
  point P16 (0.0781, -2.4988)
  point P17 (-0.1836, -2.4933)
  point P18 (-0.4432, -2.4604)
  point P19 (-0.6979, -2.4006)
  point P20 (-0.945, -2.3145)
  point P21 (-1.1818, -2.203)
  point P22 (-1.4056, -2.0674)
  point P23 (-1.614, -1.9092)
  point P24 (-1.8047, -1.73)
  point P25 (-1.9757, -1.5319)
  point P26 (-2.125, -1.317)
  point P27 (-2.251, -1.0877)
  point P28 (-2.3524, -0.8464)
  point P29 (-2.4279, -0.5959)
  point P30 (-2.4769, -0.3388)
  point P31 (-2.4988, -0.0781)
  point P32 (-2.4207, 0)
  point P33 (-2.4933, 0.1836)
  point P34 (-2.4604, 0.4432)
  point P35 (-2.4006, 0.6979)
  point P36 (-2.3145, 0.945)
  point P37 (-2.203, 1.1818)
  point P38 (-2.0674, 1.4056)
  point P39 (-1.9092, 1.614)
  point P40 (-1.73, 1.8047)
  point P41 (-1.5319, 1.9757)
  point P42 (-1.317, 2.125)
  point P43 (-1.0877, 2.251)
  point P44 (-0.8464, 2.3524)
  point P45 (-0.5959, 2.4279)
  point P46 (-0.3388, 2.4769)
  point P47 (-0.0781, 2.4988)
  point P48 (0.1836, 2.4933)
  point P49 (0.4432, 2.4604)
  point P50 (0.6979, 2.4006)
  point P51 (0.945, 2.3145)
  point P52 (1.1818, 2.203)
  point P53 (1.4056, 2.0674)
  point P54 (1.614, 1.9092)
  point P55 (1.8047, 1.73)
  point P56 (1.9757, 1.5319)
  point P57 (2.125, 1.317)
  point P58 (2.251, 1.0877)
  point P59 (2.3524, 0.8464)
  point P60 (2.4279, 0.5959)
  point P61 (2.4769, 0.3388)
  point P62 (2.4988, 0.0781)
  dimension "d0" = 0.05
  dimension "d1" = 2.498
  dimension "d2" = 1.749
  dimension "d3" = 0.05
  dimension "d4" = 2.3854
  dimension "d5" = 1.7894
  dimension "d6" = 0.05
  dimension "d7" = 0.05
  dimension "d8" = 20
  constraints: 244 end point, 120 point on circle, 61 centre point, 2 parallel, 2 point on line, 1 coincident, 183 other
  measures "d0" radial gap between concentric circles of A24 A144
  measures "d1" horizontal distance of A0.centre L244.end
  measures "d2" horizontal distance of A9.centre L195.end
  measures "d3" distance between parallel lines of L119 L238
  measures "d4" horizontal distance of A2.centre L240.end
  measures "d5" horizontal distance of point (0, 0) L242.start
  measures "d6" distance between parallel lines of L73 L241
  measures "d7" distance between parallel lines of L29 L243
  measures "d8" diameter of A204
extrude "Extrusion1" add sketch "Sketch1" along normal blind 5 contours L240 A4 L243 | L239 L238 A4 | A4 L124 L123 | L237 L236 A4 | A4 L126 L125 | L235 L234 A4 | A4 L128 L127 | L233 L232 A4 | A4 L130 L129 | L231 L230 A4 | A4 L132 L131 | L229 L228 A4 | A4 L134 L133 | L227 L226 A4 | A4 L136 L135 | L225 L224 A4 | A4 L138 L137 | L223 L222 A4 | A4 L140 L139 | L221 L220 A4 | A4 L142 L141 | L219 L218 A4 | A4 L144 L143 | L217 L216 A4 | A4 L146 L145 | L215 L214 A4 | A4 L148 L147 | L213 L212 A4 | A4 L150 L149 | L211 L210 A4 | A4 L152 L151 | L209 L208 A4 | A4 L154 L153 | L207 L206 A4 | A4 L156 L155 | L205 L204 A4 | A4 L158 L157 | L203 L202 A4 | A4 L160 L159 | L201 L200 A4 | A4 L162 L161 | L199 L198 A4 | A4 L164 L163 | L197 L196 A4 | A4 L166 L165 | L241 L195 A4 | A4 L168 L167 | L194 L193 A4 | A4 L170 L169 | L192 L191 A4 | A4 L172 L171 | L190 L189 A4 | A4 L174 L173 | L188 L187 A4 | A4 L176 L175 | L186 L185 A4 | A4 L178 L177 | L184 L183 A4 | A4 L180 L179 | L182 L181 A4 | A204
sketch "Sketch2" plane through (0, 0, 5) normal (0, 0, 1) x (1, 0, 0)
  circle A0 centre (-22.7293, 0) radius 10
  point P0 (0, 0)
  dimension "d12" = 20
  constraints: 1 centre point
  measures "d12" diameter of A0
extrude "Extrusion2" add sketch "Sketch2" against normal blind 5
body "Solid1"
